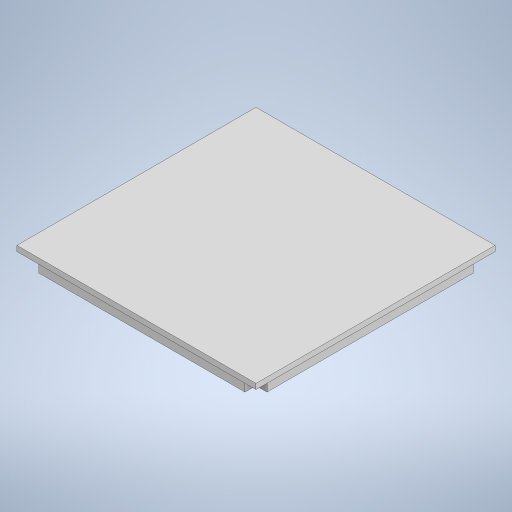
# Autodesk Inventor part: Acrilico_Bottom
Saved by Autodesk Inventor 2024 (Build 280153000, 153)
## iProperties
Created: 2023-06-25
Part Number: Acrilico_Bottom
Material: Genérico
Document SubType Name: Modeling
Designer: Personal
Density: 1 g/cm^3
Appearance: Valor por defecto
Author: Personal
Autodesk Inventor part; units mm, degrees
ref_plane "YZ Plane" through (0, 0, 0) normal (1, 0, 0) x (0, 1, 0)
ref_plane "XZ Plane" through (0, 0, 0) normal (0, 1, 0) x (-1, 0, 0)
ref_plane "XY Plane" through (0, 0, 0) normal (0, 0, 1) x (1, 0, 0)
sketch "Boceto1" plane through (0, 0, 0) normal (0, 1, 0) x (-1, 0, 0)
  line L0 (-97.5, 97.5) -> (97.5, 97.5)
  line L1 (97.5, 97.5) -> (97.5, -97.5)
  line L2 (97.5, -97.5) -> (-97.5, -97.5)
  line L3 (-97.5, -97.5) -> (-97.5, 97.5)
  line L4 (-97.5, 97.5) -> (97.5, -97.5) construction
  line L5 (97.5, 97.5) -> (-97.5, -97.5) construction
  point P0 (0, 0)
  dimension "d0" = 195
  dimension "d1" = 195
  constraints: 12 end point, 2 midpoint, 2 parallel, 1 horizontal, 1 perpendicular
  measures "d0" distance of L0.end L1.end
  measures "d1" distance of L0.start L0.end
extrude "Extrusión1" add sketch "Boceto1" along normal mid plane 4.4
sketch "Boceto4" plane through (0, -2.2, 0) normal (0, -1, 0) x (1, 0, 0)
  line L0 (97.5, -97.5) -> (97.5, 97.5) construction
  line L1 (-97.5, 97.5) -> (-97.5, -97.5) construction
  line L2 (84.1, -93.1) -> (-84.1, -93.1)
  line L3 (-84.1, -93.1) -> (-84.1, -84.1)
  line L4 (-84.1, -84.1) -> (84.1, -84.1)
  line L5 (84.1, -84.1) -> (84.1, -93.1)
  line L6 (-97.5, -97.5) -> (97.5, -97.5) construction
  line L7 (93.1, -84.1) -> (84.1, -84.1)
  line L8 (84.1, -84.1) -> (84.1, 84.1)
  line L9 (84.1, 84.1) -> (93.1, 84.1)
  line L10 (93.1, 84.1) -> (93.1, -84.1)
  line L11 (0, -126.8945) -> (0, 107.949)
  line L12 (-84.1, -84.1) -> (-84.1, 84.1)
  line L13 (-84.1, 84.1) -> (-93.1, 84.1)
  line L14 (-93.1, 84.1) -> (-93.1, -84.1)
  line L15 (-93.1, -84.1) -> (-84.1, -84.1)
  line L16 (84.1, 84.1) -> (-84.1, 84.1)
  line L17 (84.1, 93.1) -> (-84.1, 93.1)
  line L18 (84.1, 84.1) -> (84.1, 93.1)
  line L19 (-84.1, 84.1) -> (-84.1, 93.1)
  point P0 (0, 0)
  point P1 (-84.1, -88.6)
  point P2 (88.6, -84.1)
  point P3 (84.1, -84.1)
  point P4 (84.1, -84.1)
  point P5 (84.1, -84.1)
  point P6 (84.1, -84.1)
  point P7 (-84.1, 84.1)
  point P8 (-84.1, 84.1)
  point P9 (-84.1, 84.1)
  point P10 (-84.1, 84.1)
  dimension "d20" = 4.4
  dimension "d21" = 9
  dimension "d22" = 13.4
  dimension "d23" = 13.4
  dimension "d24" = 4.4
  dimension "d25" = 9
  dimension "d26" = 13.4
  dimension "d30" = 9
  constraints: 34 end point, 5 horizontal, 4 parallel, 4 symmetric about line, 3 vertical, 2 midpoint, 2 perpendicular
  measures "d20" distance between parallel lines of L2 L6
  measures "d21" distance of L4.end L2.start
  measures "d22" distance between parallel lines of L0 L5
  measures "d23" distance from line of L1 point (-84.1, -88.6)
  measures "d24" distance between parallel lines of L0 L10
  measures "d25" distance of L7.start L7.end
  measures "d26" distance from line of point (88.6, -84.1) L6
  measures "d30" distance between parallel lines of L17 L16
extrude "Extrusión6" add sketch "Boceto4" along normal blind 9 contours L2 L11 L4 L5 | L2 L3 L4 L11 | L8 L9 L10 L7 | L16 L11 L17 L18 | L15 L14 L13 L12 | L16 L19 L17 L11
sketch "Boceto5" plane through (0, -11.2, 0) normal (0, -1, 0) x (1, 0, 0)
  line L0 (-84.1, -93.1) -> (84.1, -93.1) construction
  line L1 (93.1, -84.1) -> (93.1, 84.1) construction
  line L2 (-93.1, 84.1) -> (-93.1, -84.1) construction
  line L3 (84.1, 93.1) -> (-84.1, 93.1) construction
  line L4 (84.1, -93.1) -> (-84.1, -93.1)
  line L5 (-93.1, -84.1) -> (-93.1, 84.1)
  line L6 (-84.1, 93.1) -> (84.1, 93.1)
  line L7 (93.1, 84.1) -> (93.1, -84.1)
  line L8 (84.1, -93.1) -> (84.1, -84.1) projected
  line L9 (84.1, -84.1) -> (-84.1, -84.1) construction
  line L10 (84.1, -93.1) -> (84.1, -84.1)
  line L11 (84.1, -84.1) -> (93.1, -84.1)
  line L12 (93.1, 84.1) -> (84.1, 84.1)
  line L13 (84.1, 84.1) -> (84.1, 93.1)
  line L14 (-93.1, 84.1) -> (-84.1, 84.1)
  line L15 (-84.1, 84.1) -> (-84.1, 93.1)
  line L16 (-93.1, -84.1) -> (-84.1, -84.1) projected
  line L17 (-84.1, -93.1) -> (-84.1, -84.1)
  line L18 (-84.1, -84.1) -> (-93.1, -84.1)
  point P0 (0, 0)
  constraints: 24 end point, 9 point on line, 5 perpendicular, 2 horizontal, 2 parallel, 2 vertical
extrude "Extrusión7" add sketch "Boceto5" along normal blind 1.65
